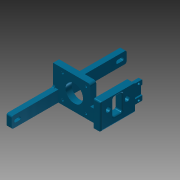
# Autodesk Inventor part: X-Axis-Stepper-Plate
Saved by Autodesk Inventor 2014 SP1 (Build 180222100, 222)
## iProperties
Created: 2016-11-26
Part Number: X-Axis-Stepper-Plate
Material: Generic
Document SubType Name: Modeling
Designer: danielsikar
Density: 1 g/cm^3
Appearance: Sky Blue Dark
Author: danielsikar
Autodesk Inventor part; units mm, degrees
ref_plane "YZ Plane" through (0, 0, 0) normal (1, 0, 0) x (0, 1, 0)
sketch "Sketch1" plane through (0, 0, 0) normal (0, 0, 1) x (1, 0, 0)
  line L0 (43.9253, 0) -> (44, 0)
  line L1 (44, 65) -> (43.9253, 65)
  line L2 (53.9253, 65) -> (63.8472, 65)
  line L3 (63.8472, 0) -> (53.9253, 0)
  line L4 (53.9253, 0) -> (43.9253, 0)
  line L5 (44, 65) -> (44, 65.0621)
  line L6 (53.9253, 65) -> (43.9253, 65)
  arc A0 (63.8472, 65) -> (63.8472, 0) centre (91, 32.5) ccw
  line L7 (44, 65) -> (0, 65)
  line L8 (0, 65) -> (0, 0)
  line L9 (0, 0) -> (44, 0)
  arc A1 (44, 65.0621) -> (43.9253, 65) centre (71, 32.5) ccw
  line L10 (28.7, 32.5) -> (137.8108, 32.5) construction
  arc A2 (44, 65.0621) -> (43.9253, 65) centre (71, 32.5) ccw construction
  arc A3 (48.298, 51.6795) -> (46.5893, 47.865) centre (86, 32.5) ccw
  line L11 (46.65, 11) -> (56.0681, 11) construction
  circle A4 centre (49.5714, 11) radius 2 construction
  circle A5 centre (49.5714, 11) radius 2
  line L12 (48.65, 49.7107) -> (40.3907, 49.7107) construction
  circle A6 centre (47.3596, 49.7107) radius 2
  arc A7 (48.298, 51.6795) -> (48.0048, 51.6038) centre (48.65, 49.7107) ccw
  dimension "d11" = 11
  dimension "d12" = 84.6
  dimension "d14" = 4
  dimension "d15" = 4
  dimension "d16" = 4
  constraints: 26 end point, 14 point on circle, 8 centre point, 8 point on line, 5 parallel, 3 horizontal, 3 perpendicular, 2 coincident, 1 collinear
  measures "d11" distance from line of L11.start L4
  measures "d12" diameter of A3
  measures "d14" diameter of A4
  measures "d15" diameter of A5
  measures "d16" diameter of A6
extrude "Extrusion1" add sketch "Sketch1" along normal blind 3 contours L9 L8 L7 L1 L6 L2 A0 L3 L4 L0
sketch "Sketch2" plane through (0, 0, 3) normal (0, 0, 1) x (1, 0, 0)
  line L0 (0, 0) -> (63.8472, 0) projected
  line L1 (10.072, 55) -> (20.072, 55)
  line L2 (20.072, 55) -> (20.072, 10)
  line L3 (20.072, 10) -> (10.072, 10)
  line L4 (10.072, 10) -> (10.072, 55)
  dimension "d19" = 10
  dimension "d20" = 45
  dimension "d21" = 10
  constraints: 8 end point, 2 parallel, 1 horizontal, 1 perpendicular
  measures "d19" distance of L2.end L3.end
  measures "d20" distance of L1.end L2.end
  measures "d21" distance between parallel lines of L0 L3
extrude "Extrusion2" add sketch "Sketch2" along normal blind 34
fillet "Fillet3" radius 1 3 edges at (10.072, 32.5, 37) (10.072, 10, 20) (10.072, 55, 20)
ref_plane "Work Plane1" through (0, 45, 0) normal (0, 1, 0) x (-1, 0, 0)
sketch "Sketch7" plane through (20.072, 7.6056, 3) normal (1, 0, 0) x (0, 0, -1)
  circle A0 centre (-21, 37.3944) radius 3
  line L0 (-6, 47.3944) -> (-28, 47.3944) projected
  line L1 (3, -7.6056) -> (3, 57.3944) projected
  circle A1 centre (-21, 12.3944) radius 3
  line L2 (-28, 2.3944) -> (-6, 2.3944) projected
  point P0 (3, -6.6056)
  dimension "d48" = 6
  dimension "d50" = 10
  dimension "d51" = 24
  dimension "d52" = 6
  dimension "d53" = 10
  constraints: 2 centre point
  measures "d48" diameter of A0
  measures "d50" distance from line of A0.centre L0
  measures "d51" distance from line of L1 A0.centre
  measures "d52" diameter of A1
  measures "d53" distance from line of A1.centre L2
extrude "Extrusion4" cut sketch "Sketch7" against normal blind 10
sketch "Sketch11" plane through (10.072, 7.6056, 3) normal (-1, 0, 0) x (0, 0, 1)
  line L0 (31, 30.8944) -> (9, 30.8944)
  line L1 (9, 30.8944) -> (9, 18.8944)
  line L2 (9, 18.8944) -> (31, 18.8944)
  line L3 (31, 18.8944) -> (31, 30.8944)
  line L4 (0, 2.3944) -> (34, 2.3944) projected
  line L5 (34, 2.3944) -> (34, 47.3944) projected
  point P0 (-3, -7.6056)
  point P1 (6, 2.3944)
  point P2 (28, 2.3944)
  point P3 (34, 8.3944)
  point P4 (34, 41.3944)
  dimension "d68" = 22
  dimension "d69" = 12
  dimension "d70" = 16.5
  dimension "d71" = 3
  constraints: 8 end point, 2 parallel, 1 horizontal, 1 perpendicular
  measures "d68" distance of L2.end L1.end
  measures "d69" distance of L1.end L0.end
  measures "d70" distance between parallel lines of L2 L4
  measures "d71" distance between parallel lines of L3 L5
extrude "Extrusion7" cut sketch "Sketch11" against normal blind 10
fillet "Fillet6" radius 2 4 edges at (15.072, 38.5, 34) (15.072, 26.5, 34) (15.072, 38.5, 12) (15.072, 26.5, 12)
fillet "Fillet7" radius 2 2 edges at (0, 0, 1.5) (0, 65, 1.5)
fillet "Fillet8" radius 2 19 edges at (10.072, 37.9142, 12.5858) (10.072, 38.5, 23) (10.072, 37.9142, 33.4142) (10.072, 32.5, 34) (10.072, 27.0858, 33.4142) (10.072, 26.5, 23) (10.072, 27.0858, 12.5858) (10.072, 32.5, 12) (20.072, 27.0858, 12.5858) (20.072, 26.5, 23) (20.072, 27.0858, 33.4142) (20.072, 32.5, 34) (20.072, 37.9142, 33.4142) (20.072, 38.5, 23) (20.072, 37.9142, 12.5858) (20.072, 32.5, 12) (0, 32.5, 3) (0.5858, 0.5858, 3) (32.9236, 0, 3)
ref_plane "Work Plane4" through (0, 20, 0) normal (0, 1, 0) x (-1, 0, 0)
sketch "Sketch16" plane through (0, 20, 0) normal (0, 1, 0) x (-1, 0, 0)
  circle A0 centre (20.928, 24) radius 11.5 projected
  circle A1 centre (5.428, 8.5) radius 1.5 projected
  circle A2 centre (5.5, 39.5) radius 1.5 projected
  circle A3 centre (36.5, 39.5) radius 1.5 projected
  circle A4 centre (36.5, 8.5) radius 1.5 projected
  line L0 (-2.072, 17.4131) -> (-8.072, 17.4131) projected
  arc A5 (-2.072, 17.4131) -> (1.928, 21.4131) centre (-2.072, 21.4131) ccw projected
  line L1 (1.928, 43) -> (1.928, 21.4131) projected
  line L2 (39.928, 43) -> (1.928, 43) projected
  line L3 (39.928, 5) -> (39.928, 43) projected
  line L4 (-8.072, 5) -> (39.928, 5) projected
  line L5 (-8.072, 17.4131) -> (-8.072, 5) projected
  line L6 (41.928, 43) -> (41.928, 5) projected
  line L7 (40, 0) -> (2, 0) projected
  line L8 (1.928, 45) -> (39.928, 45) projected
  line L9 (-0.072, 21.4131) -> (-0.072, 43) projected
  line L10 (-8.072, 19.4131) -> (-2.072, 19.4131) projected
  line L11 (-8.072, 17.4131) -> (-10.072, 17.4131) projected
  line L12 (-8.072, 17.4131) -> (-8.072, 5) projected
  line L13 (-8.072, 5) -> (-10.072, 3) projected
  line L14 (-10.072, 3) -> (-10.072, 17.4131) projected
  line L15 (-10.072, 9) -> (-10.072, 9) projected
  line L16 (-10.072, 19.4131) -> (-10.072, 3)
  line L17 (-2.072, 3) -> (-2.072, 0)
  line L18 (-2.072, 0) -> (2, 0)
  line L19 (40, 0) -> (41.928, 0)
  line L20 (41.928, 0) -> (41.928, 5)
  line L21 (-10.072, 19.4131) -> (-8.072, 19.4131)
  line L22 (-0.072, 21.4131) -> (-0.072, 19.4131)
  line L23 (-0.072, 19.4131) -> (-2.5925, 19.4131)
  line L24 (-0.072, 43) -> (-0.072, 45)
  line L25 (-0.072, 45) -> (1.928, 45)
  line L26 (39.928, 45) -> (41.928, 45)
  line L27 (41.928, 45) -> (41.928, 43)
  line L28 (-2.072, 3) -> (-10.072, 3)
  point P0 (0, 0)
  constraints: 26 end point, 8 perpendicular, 2 collinear, 1 parallel, 1 point on line, 1 vertical alignment
extrude "Extrusion10" add sketch "Sketch16" against normal blind 4
sketch "Sketch19" plane through (20.072, 7.6056, 3) normal (1, 0, 0) x (0, 0, -1)
  line L0 (-3.7088, 62.8117) -> (27.2078, 62.8117)
  line L1 (27.2078, 62.8117) -> (27.2078, -18.0977)
  line L2 (27.2078, -18.0977) -> (-3.7088, -18.0977)
  line L3 (-3.7088, -18.0977) -> (-3.7088, 62.8117)
  point P0 (3, -7.6056)
  constraints: 8 end point, 2 parallel, 1 horizontal, 1 perpendicular
extrude "Extrusion12" cut sketch "Sketch19" along normal through all
sketch "Sketch20" plane through (10.072, 11, 9) normal (-1, 0, 0) x (0, 0, 1)
  line L0 (-6, -16.1628) -> (-14.1646, -16.1628)
  line L1 (-14.1646, -16.1628) -> (-14.1646, 55.9477)
  line L2 (-14.1646, 55.9477) -> (-6, 55.9477)
  line L3 (-6, 55.9477) -> (-6, -16.1628)
  point P0 (-9, -11)
  constraints: 8 end point, 2 parallel, 1 horizontal, 1 perpendicular
extrude "Extrusion13" cut sketch "Sketch20" along normal through all both and the other way through all
sketch "Sketch22" plane through (-41.928, 16, 45) normal (-1, 0, 0) x (0, 0, 1)
  line L0 (-42, 4) -> (-42, 0) projected
  line L1 (0, 0) -> (-42, 0) projected
  line L2 (-42, 4) -> (0, 4)
  line L3 (0, 4) -> (0, 0)
  line L4 (0, 0) -> (-42, 0)
  line L5 (-42, 0) -> (-42, 4)
  point P0 (-45, -16)
  constraints: 8 end point, 2 parallel, 1 horizontal, 1 perpendicular
extrude "Extrusion15" add sketch "Sketch22" along normal blind 4
sketch "Sketch23" plane through (0, 16, 0) normal (0, -1, 0) x (1, 0, 0)
  line L0 (-45.928, 3) -> (-41.928, 3)
  line L1 (-41.928, 3) -> (-41.928, 18)
  line L2 (-41.928, 18) -> (-45.928, 18)
  line L3 (-45.928, 18) -> (-45.928, 3)
  point P0 (0, 0)
  dimension "d103" = 4
  dimension "d104" = 15
  constraints: 8 end point, 2 parallel, 1 horizontal, 1 perpendicular
  measures "d103" distance of L2.end L1.end
  measures "d104" distance of L1.end L0.end
extrude "Extrusion16" add sketch "Sketch23" along normal blind 54.5
sketch "Sketch24" plane through (0, 20, 0) normal (0, 1, 0) x (1, 0, 0)
  line L0 (-45.928, -3) -> (-41.928, -3)
  line L1 (-41.928, -3) -> (-41.928, -18)
  line L2 (-41.928, -18) -> (-45.928, -18)
  line L3 (-45.928, -18) -> (-45.928, -3)
  point P0 (0, 0)
  dimension "d107" = 4
  dimension "d108" = 15
  constraints: 8 end point, 2 parallel, 1 horizontal, 1 perpendicular
  measures "d107" distance of L1.end L2.end
  measures "d108" distance of L0.end L1.end
extrude "Extrusion17" add sketch "Sketch24" along normal blind 85
fillet "Fillet11" radius 3 2 edges at (-43.928, 105, 3) (-43.928, 105, 18)
fillet "Fillet12" radius 3 1 edges at (0.072, 18, 45)
fillet "Fillet13" radius 2 4 edges at (20.072, 10, 20) (10.3649, 10.2929, 36.7071) (15.572, 10, 37) (20.072, 32.5, 3)
fillet "Fillet14" radius 3 1 edges at (10.072, 16, 11.2065)
sketch "Sketch25" plane through (-41.928, -35.5, 3) normal (1, 0, 0) x (0, 0, -1)
  line L0 (0, -3) -> (-15, -3) projected
  arc A0 (-9.5, 1) -> (-5.5, 1) centre (-7.5, 1) ccw
  arc A1 (-5.5, 138.5) -> (-9.5, 138.5) centre (-7.5, 138.5) ccw
  line L1 (-12, 140.5) -> (-3, 140.5) projected
  arc A2 (-9.5, 135.5) -> (-5.5, 135.5) centre (-7.5, 135.5) ccw
  line L2 (-9.5, 138.5) -> (-9.5, 135.5)
  line L3 (-5.5, 135.5) -> (-5.5, 138.5)
  arc A3 (-5.5, 4) -> (-9.5, 4) centre (-7.5, 4) ccw
  line L4 (-5.5, 1) -> (-5.5, 4)
  line L5 (-9.5, 4) -> (-9.5, 1)
  point P0 (-3, -3)
  point P1 (-12, -3)
  point P2 (3, 35.5)
  dimension "d115" = 4
  dimension "d116" = 4
  dimension "d117" = 4
  dimension "d118" = 2
  dimension "d119" = 4
  dimension "d120" = 3
  dimension "d125" = 4
  dimension "d126" = 3
  constraints: 8 end point, 8 point on circle, 6 tangent, 4 centre point
  measures "d115" diameter of A0
  measures "d116" distance from line of A0.centre L0
  measures "d117" diameter of A1
  measures "d118" distance from line of L1 A1.centre
  measures "d119" diameter of A2
  measures "d120" distance of A1.centre A2.centre
  measures "d125" diameter of A3
  measures "d126" distance of A3.centre A0.centre
extrude "Extrusion19" cut sketch "Sketch25" against normal blind 50
sketch "Sketch26" plane through (20.072, 12, 37) normal (1, 0, 0) x (0, 0, -1)
  circle A0 centre (13, 8) radius 3 projected
  circle A1 centre (13, 33) radius 3 projected
  circle A2 centre (13, 33) radius 3.25
  circle A3 centre (13, 8) radius 3.25
  point P0 (37, -12)
  dimension "d127" = 6.5
  dimension "d128" = 6.5
  constraints: 2 centre point, 2 coincident
  measures "d127" diameter of A2
  measures "d128" diameter of A3
extrude "Extrusion20" cut sketch "Sketch26" against normal blind 10
sketch "Sketch27" plane through (20.072, 55, 37) normal (1, 0, 0) x (0, 0, -1)
  circle A0 centre (13, -10) radius 3.25 projected
  line L0 (32, 0) -> (0, 0) projected
  line L1 (0.9, 0) -> (25.1, 0)
  line L2 (25.1, 0) -> (25.1, 10)
  line L3 (25.1, 10) -> (0.9, 10)
  line L4 (0.9, 10) -> (0.9, 0)
  circle A1 centre (3.45, 5.4) radius 1.6
  circle A2 centre (22.55, 5.4) radius 1.6
  point P0 (34, 0)
  point P1 (37, -55)
  point P2 (2, 0)
  dimension "d131" = 24.2
  dimension "d132" = 10
  dimension "d133" = 12.1
  dimension "d134" = 3.2
  dimension "d135" = 5.4
  dimension "d136" = 9.55
  dimension "d137" = 3.2
  dimension "d138" = 9.55
  constraints: 8 end point, 2 centre point, 2 parallel, 1 horizontal, 1 perpendicular, 1 point on line
  measures "d131" distance of L3.end L2.end
  measures "d132" distance of L2.end L1.end
  measures "d133" distance from line of A0.centre L4
  measures "d134" diameter of A1
  measures "d135" distance from line of A1.centre L0
  measures "d136" horizontal distance of A0.centre A1.centre
  measures "d137" diameter of A2
  measures "d138" horizontal distance of A2.centre A0.centre
extrude "Extrusion21" add sketch "Sketch27" against normal blind 5 contours L0 L4 L3 L2
sketch "Sketch28" plane through (20.072, 12, 3) normal (1, 0, 0) x (0, 0, -1)
  circle A0 centre (-30.55, 48.4) radius 1.6 projected
  line L0 (-8.9, 53) -> (-33.1, 53) projected
  line L1 (-27, 53) -> (-15, 53)
  line L2 (-15, 53) -> (-15, 43)
  line L3 (-15, 43) -> (-27, 43)
  line L4 (-27, 43) -> (-27, 53)
  point P0 (3, -12)
  dimension "d141" = 12
  dimension "d142" = 10
  dimension "d143" = 3.55
  constraints: 8 end point, 2 parallel, 1 horizontal, 1 perpendicular, 1 point on line
  measures "d141" distance of L2.end L3.end
  measures "d142" distance of L1.end L2.end
  measures "d143" distance from line of L4 A0.centre
extrude "Extrusion22" cut sketch "Sketch28" against normal blind 2 contours L2 L3 L4 L0
fillet "Fillet16" radius 1 8 edges at (15.072, 65, 24) (15.072, 60, 11.9) (17.572, 65, 11.9) (17.572, 65, 36.1) (15.072, 60, 36.1) (15.072, 55, 24) (10.3649, 54.7071, 36.7071) (15.572, 55, 37)
sketch "Sketch31" plane through (-45.928, 16, 45) normal (-1, 0, 0) x (0, 0, 1)
  line L0 (-32.5, -47.5) -> (-32.5, -50.5) projected
  arc A0 (-36.5, -50.5) -> (-32.5, -50.5) centre (-34.5, -50.5) ccw projected
  line L1 (-36.5, -50.5) -> (-36.5, -47.5) projected
  arc A1 (-32.5, -47.5) -> (-36.5, -47.5) centre (-34.5, -47.5) ccw projected
  line L2 (-36.5, 84) -> (-36.5, 87) projected
  arc A2 (-32.5, 87) -> (-36.5, 87) centre (-34.5, 87) ccw projected
  line L3 (-32.5, 87) -> (-32.5, 84) projected
  arc A3 (-36.5, 84) -> (-32.5, 84) centre (-34.5, 84) ccw projected
  line L4 (-3, 4) -> (-3, 0) projected
  line L5 (0, 4) -> (-27, 4) projected
  arc A4 (-27, 7) -> (-24, 4) centre (-24, 7) ccw projected
  line L6 (-27, 4) -> (-27, 86) projected
  arc A5 (-27, 86) -> (-30, 89) centre (-30, 86) ccw projected
  line L7 (-39, 89) -> (-30, 89) projected
  arc A6 (-39, 89) -> (-42, 86) centre (-39, 86) ccw projected
  line L8 (-42, -54.5) -> (-42, 86) projected
  arc A7 (-42, -51.5) -> (-39, -54.5) centre (-39, -51.5) ccw projected
  line L9 (-27, -54.5) -> (-42, -54.5) projected
  arc A8 (-30, -54.5) -> (-27, -51.5) centre (-30, -51.5) ccw projected
  line L10 (-27, 0) -> (-27, -54.5) projected
  arc A9 (-24, 0) -> (-27, -3) centre (-24, -3) ccw projected
  line L11 (-27, 0) -> (0, 0) projected
  point P0 (-45, -16)
extrude "Extrusion26" add sketch "Sketch31" along normal blind 3 contours L0 A0 L1 A1 | L7 A5 L6 L5 L4 L11 L10 A8 L9 A7 L8 A6 | L2 A2 L3 A3 | A4 L5 L6 | L10 L11 A9
sketch "Sketch32" plane through (0, 20, 0) normal (0, 1, 0) x (1, 0, 0)
  arc A0 (-2.928, -45) -> (0.072, -42) centre (-2.928, -42) ccw projected
  line L0 (0.072, -42) -> (0.072, -19.4131) projected
  line L1 (0.072, -19.4131) -> (10.072, -19.4131) projected
  line L2 (10.072, -3) -> (10.072, -19.4131) projected
  line L3 (10.072, -3) -> (-41.928, -3) projected
  line L4 (-41.928, -3) -> (-41.928, -18) projected
  line L5 (-41.928, -18) -> (-45.928, -18) projected
  line L6 (-45.928, -21) -> (-45.928, -18) projected
  line L7 (-45.928, -21) -> (-48.928, -21) projected
  line L8 (-48.928, -42) -> (-48.928, -21) projected
  line L9 (-45.928, -42) -> (-48.928, -42) projected
  arc A1 (-45.928, -42) -> (-42.928, -45) centre (-42.928, -42) ccw projected
  line L10 (-45.928, -45) -> (-2.928, -45) projected
  circle A2 centre (-20.928, -24) radius 11.5 projected
  circle A3 centre (-36.5, -8.5) radius 1.5 projected
  circle A4 centre (-36.5, -39.5) radius 1.5 projected
  circle A5 centre (-5.5, -39.5) radius 1.5 projected
  circle A6 centre (-5.428, -8.5) radius 1.5 projected
  point P0 (0, 0)
extrude "Extrusion27" add sketch "Sketch32" along normal blind 4
sketch "Sketch33" plane through (-45.928, 20, 21) normal (-1, 0, 0) x (0, 0, 1)
  arc A0 (-3, 3) -> (0, 0) centre (0, 3) ccw projected
  line L0 (0, 0) -> (0, 4) projected
  line L1 (-3, 4) -> (0, 4) projected
  line L2 (-3, 3) -> (-3, 4) projected
  point P0 (-21, -20)
extrude "Extrusion28" add sketch "Sketch33" along normal blind 3
sketch "Sketch34" plane through (0, 20, 0) normal (0, 1, 0) x (1, 0, 0)
  arc A0 (-45.928, -42) -> (-42.928, -45) centre (-42.928, -42) ccw projected
  line L0 (-45.928, -45) -> (-45.928, -42) projected
  line L1 (-45.928, -45) -> (-42.928, -45) projected
  point P0 (0, 0)
extrude "Extrusion29" add sketch "Sketch34" along normal blind 4
sketch "Sketch35" plane through (-45.928, 16, 45) normal (-1, 0, 0) x (0, 0, 1)
  line L0 (-3, 8) -> (-3, 0) projected
  line L1 (-3, 0) -> (0, 0) projected
  line L2 (0, 0) -> (0, 8) projected
  line L3 (-3, 8) -> (0, 8) projected
  point P0 (-45, -16)
extrude "Extrusion30" add sketch "Sketch35" along normal blind 3
sketch "Sketch36" plane through (-45.928, 16, 45) normal (1, 0, 0) x (0, 0, -1)
  line L0 (36.5, -50.5) -> (36.5, -47.5) projected
  arc A0 (36.5, -47.5) -> (32.5, -47.5) centre (34.5, -47.5) ccw projected
  line L1 (32.5, -47.5) -> (32.5, -50.5) projected
  arc A1 (32.5, -50.5) -> (36.5, -50.5) centre (34.5, -50.5) ccw projected
  point P0 (45, -16)
extrude "Extrusion31" cut sketch "Sketch36" against normal through all
sketch "Sketch37" plane through (-45.928, 16, 45) normal (1, 0, 0) x (0, 0, -1)
  line L0 (32.5, 87) -> (32.5, 84) projected
  arc A0 (32.5, 84) -> (36.5, 84) centre (34.5, 84) ccw projected
  line L1 (36.5, 84) -> (36.5, 87) projected
  arc A1 (36.5, 87) -> (32.5, 87) centre (34.5, 87) ccw projected
  point P0 (45, -16)
extrude "Extrusion32" cut sketch "Sketch37" against normal through all
sketch "Sketch38" plane through (-45.928, 16, 45) normal (-1, 0, 0) x (0, 0, 1)
  arc A0 (-30, -54.5) -> (-27, -51.5) centre (-30, -51.5) ccw projected
  line L0 (-27, -54.5) -> (-30, -54.5) projected
  line L1 (-27, -51.5) -> (-27, -54.5) projected
  point P0 (-45, -16)
extrude "Extrusion33" add sketch "Sketch38" along normal blind 3
sketch "Sketch39" plane through (-45.928, 16, 45) normal (-1, 0, 0) x (0, 0, 1)
  arc A0 (-42, -51.5) -> (-39, -54.5) centre (-39, -51.5) ccw projected
  line L0 (-42, -54.5) -> (-42, -51.5) projected
  line L1 (-39, -54.5) -> (-42, -54.5) projected
  point P0 (-45, -16)
extrude "Extrusion34" add sketch "Sketch39" along normal blind 3
sketch "Sketch40" plane through (0, -38.5, 0) normal (0, -1, 0) x (1, 0, 0)
  line L0 (-41.928, 3) -> (-48.928, 3) projected
  line L1 (-41.928, 3) -> (-41.928, 18) projected
  line L2 (-41.928, 18) -> (-48.928, 18) projected
  line L3 (-48.928, 3) -> (-48.928, 18) projected
  point P0 (0, 0)
extrude "Extrusion35" add sketch "Sketch40" along normal blind 7.07
sketch "Sketch47" plane through (-41.928, 16, 18) normal (1, 0, 0) x (0, 0, -1)
  line L0 (5.5, -50.3679) -> (9.5, -50.3679)
  line L1 (9.5, -50.3679) -> (9.5, -58.3927)
  line L2 (9.5, -58.3927) -> (5.5, -58.3927)
  line L3 (5.5, -58.3927) -> (5.5, -50.3679)
  point P0 (18, -16)
  constraints: 8 end point, 2 parallel, 1 horizontal, 1 perpendicular
extrude "Extrusion41" cut sketch "Sketch47" against normal blind 7
sketch "Sketch48" plane through (-41.928, 16, 18) normal (1, 0, 0) x (0, 0, -1)
  line L0 (0, 0) -> (15, 0) projected
  line L1 (0, 0) -> (0, -61.57) projected
  line L2 (15, -61.57) -> (0, -61.57) projected
  line L3 (15, 0) -> (15, -61.57) projected
  line L4 (9.5, -47.5) -> (9.5, -58.3927) projected
  line L5 (9.5, -58.3927) -> (5.5, -58.3927) projected
  line L6 (5.5, -58.3927) -> (5.5, -47.5) projected
  arc A0 (9.5, -47.5) -> (5.5, -47.5) centre (7.5, -47.5) ccw projected
  line L7 (4.3327, -43.4599) -> (11.2879, -43.4599)
  line L8 (11.2879, -43.4599) -> (11.2879, -49.683)
  line L9 (11.2879, -49.683) -> (4.3327, -49.683)
  line L10 (4.3327, -49.683) -> (4.3327, -43.4599)
  point P0 (18, -16)
  constraints: 8 end point, 2 parallel, 1 horizontal, 1 perpendicular
extrude "Extrusion42" add sketch "Sketch48" against normal blind 7 contours L0 L3 L2 L1 | A0 L6 L9 L10 L7 L8 L4 | L4 L9 L6 A0
fillet "Fillet18" radius 2 4 edges at (-45.428, -42.3927, 12.5) (-45.428, -33.683, 12.5) (-45.428, -42.3927, 8.5) (-45.428, -33.683, 8.5)
sketch "Sketch50" plane through (-41.928, 100, 8.5) normal (1, 0, 0) x (0, 0, -1)
  arc A0 (0, 3) -> (-2, 5) centre (-2, 3) ccw projected
  line L0 (0, 3) -> (0, 0) projected
  arc A1 (-4, 0) -> (0, 0) centre (-2, 0) ccw projected
  line L1 (-4, 0) -> (-4, 3) projected
  arc A2 (-2, 5) -> (-4, 3) centre (-2, 3) ccw projected
  line L2 (-9.5, -76) -> (-9.5, 2) projected
  line L3 (-9.5, -2.8552) -> (5.5, -2.8552)
  line L4 (5.5, -2.8552) -> (5.5, 6.0836)
  line L5 (5.5, 6.0836) -> (-9.5, 6.0836)
  line L6 (-9.5, 6.0836) -> (-9.5, -2.8552)
  point P0 (8.5, -100)
  constraints: 8 end point, 2 parallel, 1 horizontal, 1 perpendicular, 1 point on line
extrude "Extrusion43" add sketch "Sketch50" against normal blind 7 contours L0 A1 L1 A2 A0 | L2 L6 L5 L4 L3
sketch "Sketch51" plane through (-41.928, 24, 18) normal (1, 0, 0) x (0, 0, -1)
  line L0 (5.25, 68.3482) -> (9.75, 68.3482)
  line L1 (9.75, 68.3482) -> (9.75, 78.5737)
  line L2 (9.75, 78.5737) -> (5.25, 78.5737)
  line L3 (5.25, 78.5737) -> (5.25, 68.3482)
  point P0 (18, -24)
  constraints: 8 end point, 2 parallel, 1 horizontal, 1 perpendicular
extrude "Extrusion44" cut sketch "Sketch51" against normal blind 7
fillet "Fillet19" radius 2 4 edges at (-45.428, 92.3482, 8.25) (-45.428, 102.5737, 8.25) (-45.428, 102.5737, 12.75) (-45.428, 92.3482, 12.75)
fillet "Fillet20" radius 2 4 edges at (-45.428, -45.57, 3) (-45.428, -45.57, 18) (-45.428, 106.0836, 18) (-45.428, 106.0836, 3)
body "Solid1"
